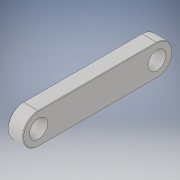
# Autodesk Inventor part: Reverse Gear Drag Link
Saved by Autodesk Inventor 2017 (Build 210142000, 142)
## iProperties
Created: 2018-10-30
Part Number: Reverse Gear Drag Link
Material: Generic
Document SubType Name: Modeling
Designer: 623516
Density: 1 g/cm^3
Appearance: Default
Author: 623516
Autodesk Inventor part; units mm, degrees
ref_plane "YZ Plane" through (0, 0, 0) normal (1, 0, 0) x (0, 1, 0)
ref_plane "XZ Plane" through (0, 0, 0) normal (0, 1, 0) x (-1, 0, 0)
ref_plane "XY Plane" through (0, 0, 0) normal (0, 0, 1) x (1, 0, 0)
sketch "Sketch1" plane through (0, 0, 0) normal (1, 0, 0) x (0, 1, 0)
  line L0 (6, 0) -> (6, -23)
  line L1 (0, -23) -> (0, 0)
  arc A0 (6, 0) -> (0, 0) centre (3, 0) ccw
  arc A1 (0, -23) -> (6, -23) centre (3, -23) ccw
  circle A2 centre (3, 0) radius 1.75
  circle A3 centre (3, -23) radius 1.75
  dimension "d0" = 6
  dimension "d1" = 23
  dimension "d2" = 3
  dimension "d3" = 3
  dimension "d4" = 3.5
  dimension "d5" = 3.5
  constraints: 4 centre point, 4 end point, 4 point on circle, 2 coincident, 2 tangent, 1 parallel, 1 vertical
  measures "d0" distance of L0.end L1.start
  measures "d1" distance of L0.start L0.end
  measures "d2" radius of A0
  measures "d3" radius of A1
  measures "d4" diameter of A2
  measures "d5" diameter of A3
extrude "Extrusion1" add sketch "Sketch1" along normal blind 3
fillet "Fillet1" radius 0.1 8 edges at (3, 3, 3) (3, 0, -11.5) (3, 3, -26) (3, 6, -11.5) (0, 3, 3) (0, 0, -11.5) (0, 3, -26) (0, 6, -11.5)
body "Solid1"
